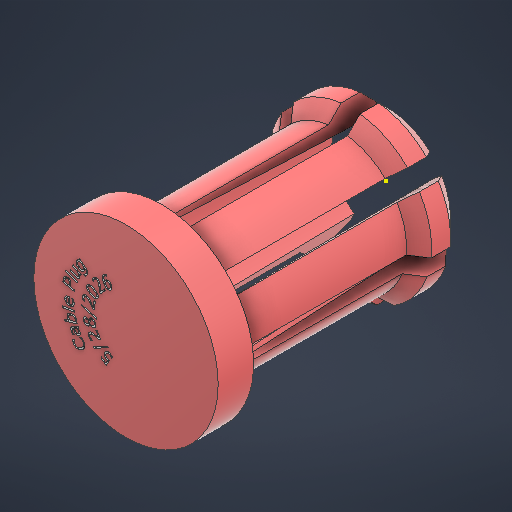
# Autodesk Inventor part: WirePlugs
Saved by Autodesk Inventor 2026.2 (Build 302298000, 298)
## iProperties
Created: 2026-05-27
Part Number: WirePlugs
Material: Generic
Document SubType Name: Modeling
Designer: mayhe
Density: 1 g/cm^3
Appearance: Default
Author: mayhe
Autodesk Inventor part; units mm, degrees
ref_plane "YZ Plane" through (0, 0, 0) normal (1, 0, 0) x (0, 1, 0)
ref_plane "XZ Plane" through (0, 0, 0) normal (0, 1, 0) x (-1, 0, 0)
ref_plane "XY Plane" through (0, 0, 0) normal (0, 0, 1) x (1, 0, 0)
sketch "Sketch1" plane through (0, 0, 0) normal (0, 0, 1) x (1, 0, 0)
  circle A0 centre (0, 0) radius 19.5
  dimension "d0" = 39
  constraints: 1 centre point, 1 coincident
  measures "d0" diameter of A0
extrude "Body" add sketch "Sketch1" along normal mid plane 55
sketch "Sketch2" plane through (0, 0, -27.5) normal (0, 0, -1) x (-1, 0, 0)
  point P0 (0, 0)
sketch "Sketch3" plane through (0, 0, 0) normal (1, 0, 0) x (0, 1, 0)
  line L0 (19.5, 20) -> (14.5, 20)
  line L1 (14.5, 20) -> (14.5, -20)
  line L2 (14.5, -20) -> (17.15, -20)
  line L3 (17.15, -20) -> (17.15, -27.5)
  line L4 (-19.5, -27.5) -> (19.5, -27.5) projected
  line L5 (19.5, 20) -> (19.5, -27.5)
  line L6 (17.15, -27.5) -> (19.5, -27.5)
  line L7 (0, -38.5) -> (0, 38.5) projected
  line L8 (19.5, 27.5) -> (-19.5, 27.5) projected
  point P0 (0, 0)
  dimension "d4" = 5
  dimension "d5" = 40
  dimension "d6" = 2.65
  dimension "d27" = 7.5
  constraints: 12 end point, 3 perpendicular, 1 collinear, 1 horizontal, 1 point on line
  measures "d4" distance of L0.start L0.end
  measures "d5" distance of L0.end L1.end
  measures "d6" distance of L1.end L2.end
  measures "d27" distance from line of L8 L0.start
revolve "Revolution1" cut sketch "Sketch3" angle 360 about axis through (0, 0, -10) along (0, 0, 1)
chamfer "Chamfer1" distance 3.5 angle 45 1 edges at (0, -17.15, -27.5)
chamfer "Chamfer2" distance 2.65 angle 45 1 edges at (0, -14.5, -20)
sketch "Sketch4" plane through (0, 0, -27.5) normal (0, 0, -1) x (-1, 0, 0)
  circle A0 centre (0, 0) radius 11.5
  dimension "d14" = 23
  constraints: 1 centre point, 1 coincident
  measures "d14" diameter of A0
extrude "Extrusion2" cut sketch "Sketch4" against normal up to surface (47.5 mm away) draft 2.5
sketch "Sketch5" plane through (0, 0, -27.5) normal (0, 0, -1) x (-1, 0, 0)
  line L0 (-2, 18.114) -> (2, 18.114)
  line L1 (2, 18.114) -> (2, 9.186)
  line L2 (2, 9.186) -> (-2, 9.186)
  line L3 (-2, 9.186) -> (-2, 18.114)
  circle A0 centre (0, 0) radius 13.65 projected
  line L4 (-2, 18.114) -> (2, 9.186) construction
  line L5 (2, 18.114) -> (-2, 9.186) construction
  line L6 (-15.4091, 9.7302) -> (-12.9151, 12.8576)
  line L7 (-12.9151, 12.8576) -> (-8.4289, 4.1637) construction
  line L8 (-12.9151, 12.8576) -> (-5.9349, 7.291)
  line L9 (-15.4091, 9.7302) -> (-5.9349, 7.291) construction
  line L10 (-8.4289, 4.1637) -> (-15.4091, 9.7302)
  line L11 (-5.9349, 7.291) -> (-8.4289, 4.1637)
  line L12 (-17.2148, -5.9806) -> (-18.1049, -2.0809)
  line L13 (-18.1049, -2.0809) -> (-8.5106, -3.9939) construction
  line L14 (-18.1049, -2.0809) -> (-9.4007, -0.0942)
  line L15 (-17.2148, -5.9806) -> (-9.4007, -0.0942) construction
  line L16 (-8.5106, -3.9939) -> (-17.2148, -5.9806)
  line L17 (-9.4007, -0.0942) -> (-8.5106, -3.9939)
  line L18 (-6.0574, -17.1879) -> (-9.6613, -15.4524)
  line L19 (-9.6613, -15.4524) -> (-2.1837, -9.144) construction
  line L20 (-9.6613, -15.4524) -> (-5.7876, -7.4085)
  line L21 (-6.0574, -17.1879) -> (-5.7876, -7.4085) construction
  line L22 (-2.1837, -9.144) -> (-6.0574, -17.1879)
  line L23 (-5.7876, -7.4085) -> (-2.1837, -9.144)
  line L24 (9.6613, -15.4524) -> (6.0574, -17.1879)
  line L25 (6.0574, -17.1879) -> (5.7876, -7.4085) construction
  line L26 (6.0574, -17.1879) -> (2.1837, -9.144)
  line L27 (9.6613, -15.4524) -> (2.1837, -9.144) construction
  line L28 (5.7876, -7.4085) -> (9.6613, -15.4524)
  line L29 (2.1837, -9.144) -> (5.7876, -7.4085)
  line L30 (18.1049, -2.0809) -> (17.2148, -5.9806)
  line L31 (17.2148, -5.9806) -> (9.4007, -0.0942) construction
  line L32 (17.2148, -5.9806) -> (8.5106, -3.9939)
  line L33 (18.1049, -2.0809) -> (8.5106, -3.9939) construction
  line L34 (9.4007, -0.0942) -> (18.1049, -2.0809)
  line L35 (8.5106, -3.9939) -> (9.4007, -0.0942)
  line L36 (12.9151, 12.8576) -> (15.4091, 9.7302)
  line L37 (15.4091, 9.7302) -> (5.9349, 7.291) construction
  line L38 (15.4091, 9.7302) -> (8.4289, 4.1637)
  line L39 (12.9151, 12.8576) -> (8.4289, 4.1637) construction
  line L40 (5.9349, 7.291) -> (12.9151, 12.8576)
  line L41 (8.4289, 4.1637) -> (5.9349, 7.291)
  point P0 (0, 13.65)
  point P1 (-10.672, 8.5106)
  point P2 (-13.3078, -3.0374)
  point P3 (-5.9225, -12.2982)
  point P4 (5.9225, -12.2982)
  point P5 (13.3078, -3.0374)
  point P6 (10.672, 8.5106)
  dimension "d17" = 4
  dimension "d20" = 360
  constraints: 84 end point, 2 midpoint, 2 parallel, 1 horizontal, 1 perpendicular, 1 vertical alignment, 79 other
  measures "d17" distance of L1.end L2.end
extrude "Extrusion3" cut sketch "Sketch5" against normal up to surface (47.5 mm away) contours L0 L1 A0 L3 | A0 L1 L2 L3 | L8 L11 L10 A0 | A0 L10 L6 L8 | L40 L36 L38 A0 | A0 L38 L41 L40 | L14 L17 L16 A0 | A0 L16 L12 L14 | L34 L30 L32 A0 | A0 L32 L35 L34 | L20 L23 L22 A0 | A0 L22 L18 L20 | L28 L24 L26 A0 | A0 L26 L29 L28
chamfer "Chamfer3" distance 1 angle 45 14 edges at (-2, 13.8936, 20) (2, 13.8936, 20) (9.6155, 10.2262, 20) (12.1094, 7.0988, 20) (13.9903, -1.1418, 20) (13.1002, -5.0415, 20) (7.8301, -11.6499, 20) (4.2263, -13.3854, 20) (-4.2263, -13.3854, 20) (-7.8301, -11.6499, 20) (-13.1002, -5.0415, 20) (-13.9903, -1.1418, 20) (-12.1094, 7.0988, 20) (-9.6155, 10.2262, 20)
sketch "Sketch6" plane through (0, 0, 27.5) normal (0, 0, 1) x (1, 0, 0)
  circle A0 centre (0, 0) radius 11
  spline S0 degree 2 poles (-8.9107, -6.3753) (-8.7634, -6.5735) (-8.6478, -7.0083) (-8.6908, -7.23) knots 0 0 0 1 2 2 2
  spline S1 degree 2 poles (-8.6908, -7.23) (-8.732, -7.4505) (-9.029, -7.8791) (-9.2866, -8.0707) knots 0 0 0 1 2 2 2
  spline S2 degree 2 poles (-9.2866, -8.0707) (-9.5427, -8.261) (-10.0196, -8.413) (-10.2521, -8.3935) knots 0 0 0 1 2 2 2
  spline S3 degree 2 poles (-10.2521, -8.3935) (-10.4801, -8.3732) (-10.8719, -8.1464) (-11.0254, -7.94) knots 0 0 0 1 2 2 2
  spline S4 degree 2 poles (-11.0254, -7.94) (-11.1016, -7.8375) (-11.2057, -7.6354) (-11.2391, -7.5422) knots 0 0 0 1 2 2 2
  spline S5 degree 2 poles (-11.2391, -7.5422) (-11.2667, -7.4602) (-11.3075, -7.2776) (-11.3216, -7.1829) knots 0 0 0 1 2 2 2
  line L0 (-11.3216, -7.1829) -> (-10.9945, -6.9397)
  line L1 (-10.9945, -6.9397) -> (-10.9785, -6.9612)
  spline S6 degree 2 poles (-10.9785, -6.9612) (-10.9846, -7.0221) (-10.9935, -7.2032) (-10.978, -7.3173) knots 0 0 0 1 2 2 2
  spline S7 degree 2 poles (-10.978, -7.3173) (-10.9632, -7.4269) (-10.8814, -7.6507) (-10.7929, -7.7697) knots 0 0 0 1 2 2 2
  spline S8 degree 2 poles (-10.7929, -7.7697) (-10.6959, -7.9002) (-10.4154, -8.0532) (-10.2479, -8.0646) knots 0 0 0 1 2 2 2
  spline S9 degree 2 poles (-10.2479, -8.0646) (-10.0799, -8.0731) (-9.6932, -7.9344) (-9.4967, -7.7882) knots 0 0 0 1 2 2 2
  spline S10 degree 2 poles (-9.4967, -7.7882) (-9.2869, -7.6322) (-9.0595, -7.3067) (-9.0206, -7.1418) knots 0 0 0 1 2 2 2
  spline S11 degree 2 poles (-9.0206, -7.1418) (-8.9837, -6.981) (-9.052, -6.6753) (-9.1478, -6.5464) knots 0 0 0 1 2 2 2
  spline S12 degree 2 poles (-9.1478, -6.5464) (-9.235, -6.4291) (-9.4414, -6.2723) (-9.542, -6.2266) knots 0 0 0 1 2 2 2
  spline S13 degree 2 poles (-9.542, -6.2266) (-9.6403, -6.1842) (-9.8117, -6.1398) (-9.8665, -6.1318) knots 0 0 0 1 2 2 2
  line L2 (-9.8665, -6.1318) -> (-9.8812, -6.1119)
  line L3 (-9.8812, -6.1119) -> (-9.5574, -5.8712)
  spline S14 degree 2 poles (-9.5574, -5.8712) (-9.4757, -5.9156) (-9.3295, -5.9915) (-9.2404, -6.0561) knots 0 0 0 1 2 2 2
  spline S15 degree 2 poles (-9.2404, -6.0561) (-9.1444, -6.1232) (-9.0016, -6.2531) (-8.9107, -6.3753) knots 0 0 0 1 2 2 2
  spline S16 degree 2 poles (-10.1998, -4.646) (-10.1566, -4.6682) (-10.0058, -4.7404) (-9.9507, -4.782) knots 0 0 0 1 2 2 2
  spline S17 degree 2 poles (-9.9507, -4.782) (-9.8726, -4.8374) (-9.7596, -4.9583) (-9.6955, -5.0873) knots 0 0 0 1 2 2 2
  spline S18 degree 2 poles (-9.6955, -5.0873) (-9.6433, -5.1924) (-9.6283, -5.4216) (-9.6644, -5.5292) knots 0 0 0 1 2 2 2
  spline S19 degree 2 poles (-9.6644, -5.5292) (-9.7006, -5.6322) (-9.8658, -5.8178) (-9.9801, -5.8745) knots 0 0 0 1 2 2 2
  spline S20 degree 2 poles (-9.9801, -5.8745) (-10.1571, -5.9625) (-10.482, -5.9377) (-10.6345, -5.8112) knots 0 0 0 1 2 2 2
  spline S21 degree 2 poles (-10.6345, -5.8112) (-10.7723, -5.7004) (-11.0162, -5.3343) (-11.1417, -5.114) knots 0 0 0 1 2 2 2
  line L4 (-11.1417, -5.114) -> (-11.197, -5.1415)
  spline S22 degree 2 poles (-11.197, -5.1415) (-11.2966, -5.191) (-11.3899, -5.3132) (-11.3974, -5.3859) knots 0 0 0 1 2 2 2
  spline S23 degree 2 poles (-11.3974, -5.3859) (-11.405, -5.4586) (-11.3483, -5.6281) (-11.3062, -5.7129) knots 0 0 0 1 2 2 2
  spline S24 degree 2 poles (-11.3062, -5.7129) (-11.2567, -5.8124) (-11.064, -6.0522) (-10.94, -6.1584) knots 0 0 0 1 2 2 2
  line L5 (-10.94, -6.1584) -> (-10.9318, -6.175)
  line L6 (-10.9318, -6.175) -> (-11.2249, -6.3206)
  spline S25 degree 2 poles (-11.2249, -6.3206) (-11.2864, -6.2523) (-11.4891, -5.983) (-11.5615, -5.8374) knots 0 0 0 1 2 2 2
  spline S26 degree 2 poles (-11.5615, -5.8374) (-11.6494, -5.6605) (-11.7141, -5.3915) (-11.6898, -5.2599) knots 0 0 0 1 2 2 2
  spline S27 degree 2 poles (-11.6898, -5.2599) (-11.6665, -5.1311) (-11.4892, -4.9281) (-11.3289, -4.8484) knots 0 0 0 1 2 2 2
  line L7 (-11.3289, -4.8484) -> (-10.162, -4.2687)
  line L8 (-10.162, -4.2687) -> (-10.0191, -4.5563)
  line L9 (-10.0191, -4.5563) -> (-10.1998, -4.646)
  line L10 (-10.4394, -4.7651) -> (-10.9132, -5.0005)
  spline S28 degree 2 poles (-10.9132, -5.0005) (-10.8527, -5.0991) (-10.6665, -5.3951) (-10.5885, -5.4781) knots 0 0 0 1 2 2 2
  spline S29 degree 2 poles (-10.5885, -5.4781) (-10.4967, -5.575) (-10.2769, -5.652) (-10.1479, -5.5878) knots 0 0 0 1 2 2 2
  spline S30 degree 2 poles (-10.1479, -5.5878) (-10.0004, -5.5146) (-9.9335, -5.2745) (-10.0123, -5.116) knots 0 0 0 1 2 2 2
  spline S31 degree 2 poles (-10.0123, -5.116) (-10.0791, -4.9814) (-10.3052, -4.8179) (-10.4394, -4.7651) knots 0 0 0 1 2 2 2
  spline S32 degree 2 poles (-11.7296, -2.6033) (-11.2819, -2.4695) (-10.606, -2.7401) (-10.5081, -3.0675) knots 0 0 0 1 2 2 2
  spline S33 degree 2 poles (-10.5081, -3.0675) (-10.4639, -3.2154) (-10.4738, -3.4482) (-10.5063, -3.5697) knots 0 0 0 1 2 2 2
  line L11 (-10.5063, -3.5697) -> (-10.4156, -3.564)
  line L12 (-10.4156, -3.564) -> (-10.3295, -3.852)
  line L13 (-10.3295, -3.852) -> (-12.8716, -4.6117)
  line L14 (-12.8716, -4.6117) -> (-12.9636, -4.3041)
  line L15 (-12.9636, -4.3041) -> (-12.0564, -4.0329)
  spline S34 degree 2 poles (-12.0564, -4.0329) (-12.1957, -3.9478) (-12.4145, -3.7189) (-12.4658, -3.5473) knots 0 0 0 1 2 2 2
  spline S35 degree 2 poles (-12.4658, -3.5473) (-12.5583, -3.2377) (-12.1694, -2.7348) (-11.7296, -2.6033) knots 0 0 0 1 2 2 2
  spline S36 degree 2 poles (-11.611, -2.9138) (-11.9384, -3.0116) (-12.2181, -3.3122) (-12.1521, -3.5331) knots 0 0 0 1 2 2 2
  spline S37 degree 2 poles (-12.1521, -3.5331) (-12.115, -3.6573) (-11.92, -3.8783) (-11.798, -3.9557) knots 0 0 0 1 2 2 2
  line L16 (-11.798, -3.9557) -> (-10.7508, -3.6427)
  spline S38 degree 2 poles (-10.7508, -3.6427) (-10.7284, -3.5093) (-10.7347, -3.3157) (-10.7665, -3.2092) knots 0 0 0 1 2 2 2
  spline S39 degree 2 poles (-10.7665, -3.2092) (-10.8367, -2.9745) (-11.2501, -2.8059) (-11.611, -2.9138) knots 0 0 0 1 2 2 2
  line L17 (-10.8743, -1.6658) -> (-10.8211, -1.9824)
  line L18 (-10.8211, -1.9824) -> (-13.4376, -2.4224)
  line L19 (-13.4376, -2.4224) -> (-13.4908, -2.1057)
  line L20 (-13.4908, -2.1057) -> (-10.8743, -1.6658)
  spline S40 degree 2 poles (-10.9513, -0.3734) (-10.9299, -0.8299) (-11.4183, -1.3556) (-11.8912, -1.3778) knots 0 0 0 1 2 2 2
  spline S41 degree 2 poles (-11.8912, -1.3778) (-12.3558, -1.3997) (-12.9298, -0.9383) (-12.9482, -0.5456) knots 0 0 0 1 2 2 2
  spline S42 degree 2 poles (-12.9482, -0.5456) (-12.9565, -0.3687) (-12.8666, -0.0905) (-12.7623, 0.0154) knots 0 0 0 1 2 2 2
  spline S43 degree 2 poles (-12.7623, 0.0154) (-12.6582, 0.1233) (-12.3487, 0.2471) (-12.1205, 0.2578) knots 0 0 0 1 2 2 2
  line L21 (-12.1205, 0.2578) -> (-11.9457, 0.266)
  line L22 (-11.9457, 0.266) -> (-11.8838, -1.0519)
  spline S44 degree 2 poles (-11.8838, -1.0519) (-11.5528, -1.0364) (-11.2168, -0.6868) (-11.2308, -0.3907) knots 0 0 0 1 2 2 2
  spline S45 degree 2 poles (-11.2308, -0.3907) (-11.2357, -0.2858) (-11.2925, -0.0845) (-11.3334, -0.004) knots 0 0 0 1 2 2 2
  spline S46 degree 2 poles (-11.3334, -0.004) (-11.3786, 0.0804) (-11.4562, 0.1963) (-11.4909, 0.2338) knots 0 0 0 1 2 2 2
  line L23 (-11.4909, 0.2338) -> (-11.4918, 0.2523)
  line L24 (-11.4918, 0.2523) -> (-11.1422, 0.2688)
  spline S47 degree 2 poles (-11.1422, 0.2688) (-11.117, 0.2143) (-11.0433, 0.0488) (-11.0217, -0.0161) knots 0 0 0 1 2 2 2
  spline S48 degree 2 poles (-11.0217, -0.0161) (-10.9906, -0.1074) (-10.9567, -0.2583) (-10.9513, -0.3734) knots 0 0 0 1 2 2 2
  spline S49 degree 2 poles (-12.1757, -0.058) (-12.3051, -0.0682) (-12.4917, -0.1305) (-12.553, -0.1849) knots 0 0 0 1 2 2 2
  spline S50 degree 2 poles (-12.553, -0.1849) (-12.6224, -0.2438) (-12.6902, -0.4222) (-12.6842, -0.5517) knots 0 0 0 1 2 2 2
  spline S51 degree 2 poles (-12.6842, -0.5517) (-12.6782, -0.6792) (-12.5937, -0.8545) (-12.5162, -0.925) knots 0 0 0 1 2 2 2
  spline S52 degree 2 poles (-12.5162, -0.925) (-12.4367, -0.9934) (-12.2503, -1.0588) (-12.1285, -1.0634) knots 0 0 0 1 2 2 2
  line L25 (-12.1285, -1.0634) -> (-12.1757, -0.058)
  spline S53 degree 2 poles (-12.2596, 3.7005) (-12.099, 3.6641) (-11.8359, 3.4841) (-11.7587, 3.359) knots 0 0 0 1 2 2 2
  spline S54 degree 2 poles (-11.7587, 3.359) (-11.6614, 3.2019) (-11.6096, 2.825) (-11.6696, 2.56) knots 0 0 0 1 2 2 2
  line L26 (-11.6696, 2.56) -> (-11.7328, 2.281)
  line L27 (-11.7328, 2.281) -> (-10.8094, 2.0717)
  line L28 (-10.8094, 2.0717) -> (-10.884, 1.7425)
  line L29 (-10.884, 1.7425) -> (-13.3612, 2.3039)
  line L30 (-13.3612, 2.3039) -> (-13.2202, 2.9262)
  spline S55 degree 2 poles (-13.2202, 2.9262) (-13.1702, 3.147) (-13.0278, 3.4398) (-12.9187, 3.5396) knots 0 0 0 1 2 2 2
  spline S56 degree 2 poles (-12.9187, 3.5396) (-12.7929, 3.6567) (-12.4664, 3.7473) (-12.2596, 3.7005) knots 0 0 0 1 2 2 2
  spline S57 degree 2 poles (-12.3274, 3.3549) (-12.4558, 3.384) (-12.6646, 3.3385) (-12.7453, 3.2618) knots 0 0 0 1 2 2 2
  spline S58 degree 2 poles (-12.7453, 3.2618) (-12.8152, 3.1953) (-12.9047, 2.9961) (-12.9397, 2.8415) knots 0 0 0 1 2 2 2
  line L31 (-12.9397, 2.8415) -> (-13.0016, 2.5685)
  line L32 (-13.0016, 2.5685) -> (-12.0139, 2.3447)
  line L33 (-12.0139, 2.3447) -> (-11.9629, 2.5695)
  spline S59 degree 2 poles (-11.9629, 2.5695) (-11.9175, 2.7703) (-11.9257, 3.0317) (-11.9919, 3.1311) knots 0 0 0 1 2 2 2
  spline S60 degree 2 poles (-11.9919, 3.1311) (-12.0493, 3.2223) (-12.2089, 3.3281) (-12.3274, 3.3549) knots 0 0 0 1 2 2 2
  line L34 (-10.2918, 3.8865) -> (-10.4008, 3.5845)
  line L35 (-10.4008, 3.5845) -> (-12.8964, 4.4855)
  line L36 (-12.8964, 4.4855) -> (-12.7873, 4.7875)
  line L37 (-12.7873, 4.7875) -> (-10.2918, 3.8865)
  line L38 (-9.4657, 5.6523) -> (-9.6115, 5.3662)
  line L39 (-9.6115, 5.3662) -> (-9.7986, 5.4615)
  spline S61 degree 2 poles (-9.7986, 5.4615) (-9.7503, 5.2706) (-9.7515, 4.9732) (-9.8263, 4.8265) knots 0 0 0 1 2 2 2
  spline S62 degree 2 poles (-9.8263, 4.8265) (-9.8823, 4.7165) (-10.0556, 4.5576) (-10.1709, 4.5262) knots 0 0 0 1 2 2 2
  spline S63 degree 2 poles (-10.1709, 4.5262) (-10.2872, 4.493) (-10.5685, 4.5347) (-10.741, 4.6225) knots 0 0 0 1 2 2 2
  line L40 (-10.741, 4.6225) -> (-11.8433, 5.1839)
  line L41 (-11.8433, 5.1839) -> (-11.6976, 5.47)
  line L42 (-11.6976, 5.47) -> (-10.7291, 4.9768)
  spline S64 degree 2 poles (-10.7291, 4.9768) (-10.5934, 4.9077) (-10.4052, 4.8372) (-10.3214, 4.8385) knots 0 0 0 1 2 2 2
  spline S65 degree 2 poles (-10.3214, 4.8385) (-10.2377, 4.8397) (-10.1164, 4.9281) (-10.0594, 5.04) knots 0 0 0 1 2 2 2
  spline S66 degree 2 poles (-10.0594, 5.04) (-10.0062, 5.1445) (-10.0049, 5.4418) (-10.0407, 5.5848) knots 0 0 0 1 2 2 2
  line L43 (-10.0407, 5.5848) -> (-11.3099, 6.2312)
  line L44 (-11.3099, 6.2312) -> (-11.1642, 6.5173)
  line L45 (-11.1642, 6.5173) -> (-9.4657, 5.6523)
  spline S67 degree 2 poles (-8.9354, 5.9154) (-8.904, 5.933) (-8.7922, 6.0059) (-8.729, 6.0588) knots 0 0 0 1 2 2 2
  spline S68 degree 2 poles (-8.729, 6.0588) (-8.6576, 6.1158) (-8.5457, 6.2196) (-8.4924, 6.2902) knots 0 0 0 1 2 2 2
  spline S69 degree 2 poles (-8.4924, 6.2902) (-8.4031, 6.4085) (-8.3414, 6.6198) (-8.3625, 6.708) knots 0 0 0 1 2 2 2
  spline S70 degree 2 poles (-8.3625, 6.708) (-8.3849, 6.7945) (-8.505, 6.9394) (-8.5986, 7.0102) knots 0 0 0 1 2 2 2
  line L46 (-8.5986, 7.0102) -> (-8.7317, 7.1106)
  spline S71 degree 2 poles (-8.7317, 7.1106) (-8.7195, 6.9389) (-8.7842, 6.6757) (-8.8971, 6.5262) knots 0 0 0 1 2 2 2
  spline S72 degree 2 poles (-8.8971, 6.5262) (-9.0931, 6.2667) (-9.7111, 6.2511) (-10.0741, 6.5252) knots 0 0 0 1 2 2 2
  spline S73 degree 2 poles (-10.0741, 6.5252) (-10.2629, 6.6679) (-10.4747, 6.9955) (-10.5112, 7.1623) knots 0 0 0 1 2 2 2
  spline S74 degree 2 poles (-10.5112, 7.1623) (-10.5436, 7.3209) (-10.4729, 7.6364) (-10.3787, 7.7613) knots 0 0 0 1 2 2 2
  spline S75 degree 2 poles (-10.3787, 7.7613) (-10.2893, 7.8795) (-10.1032, 8.0098) (-9.9866, 8.0584) knots 0 0 0 1 2 2 2
  line L47 (-9.9866, 8.0584) -> (-10.0395, 8.1216)
  line L48 (-10.0395, 8.1216) -> (-9.8571, 8.363)
  line L49 (-9.8571, 8.363) -> (-8.5102, 7.3458)
  spline S76 degree 2 poles (-8.5102, 7.3458) (-8.1226, 7.053) (-8.0156, 6.4434) (-8.2773, 6.0968) knots 0 0 0 1 2 2 2
  spline S77 degree 2 poles (-8.2773, 6.0968) (-8.3617, 5.9851) (-8.574, 5.7792) (-8.6792, 5.7013) knots 0 0 0 1 2 2 2
  line L50 (-8.6792, 5.7013) -> (-8.9453, 5.9023)
  line L51 (-8.9453, 5.9023) -> (-8.9354, 5.9154)
  line L52 (-8.9419, 7.2694) -> (-9.778, 7.9009)
  spline S78 degree 2 poles (-9.778, 7.9009) (-9.8959, 7.8403) (-10.0569, 7.7091) (-10.1177, 7.6286) knots 0 0 0 1 2 2 2
  spline S79 degree 2 poles (-10.1177, 7.6286) (-10.2641, 7.4348) (-10.147, 6.9956) (-9.8793, 6.7934) knots 0 0 0 1 2 2 2
  spline S80 degree 2 poles (-9.8793, 6.7934) (-9.6263, 6.6023) (-9.2341, 6.5718) (-9.0902, 6.7623) knots 0 0 0 1 2 2 2
  spline S81 degree 2 poles (-9.0902, 6.7623) (-9.0145, 6.8625) (-8.9346, 7.1323) (-8.9419, 7.2694) knots 0 0 0 1 2 2 2
  spline S82 degree 2 poles (-4.4923, -6.1203) (-4.3995, -5.9624) (-4.1398, -5.7521) (-3.9892, -5.707) knots 0 0 0 1 2 2 2
  spline S83 degree 2 poles (-3.9892, -5.707) (-3.8385, -5.6618) (-3.4956, -5.7081) (-3.3253, -5.8082) knots 0 0 0 1 2 2 2
  spline S84 degree 2 poles (-3.3253, -5.8082) (-3.1691, -5.9) (-2.9046, -6.1486) (-2.8251, -6.2693) knots 0 0 0 1 2 2 2
  line L53 (-2.8251, -6.2693) -> (-3.0076, -6.5799)
  line L54 (-3.0076, -6.5799) -> (-3.0289, -6.5674)
  spline S85 degree 2 poles (-3.0289, -6.5674) (-3.048, -6.5227) (-3.1365, -6.3848) (-3.1961, -6.3115) knots 0 0 0 1 2 2 2
  spline S86 degree 2 poles (-3.1961, -6.3115) (-3.2653, -6.2303) (-3.3892, -6.1121) (-3.4797, -6.0589) knots 0 0 0 1 2 2 2
  spline S87 degree 2 poles (-3.4797, -6.0589) (-3.5685, -6.0067) (-3.7728, -5.9726) (-3.8738, -6.0063) knots 0 0 0 1 2 2 2
  spline S88 degree 2 poles (-3.8738, -6.0063) (-3.9674, -6.0397) (-4.1264, -6.1802) (-4.1953, -6.2973) knots 0 0 0 1 2 2 2
  spline S89 degree 2 poles (-4.1953, -6.2973) (-4.2641, -6.4144) (-4.2878, -6.601) (-4.2567, -6.6862) knots 0 0 0 1 2 2 2
  spline S90 degree 2 poles (-4.2567, -6.6862) (-4.2269, -6.7777) (-4.0695, -6.9323) (-3.9577, -6.998) knots 0 0 0 1 2 2 2
  spline S91 degree 2 poles (-3.9577, -6.998) (-3.837, -7.0689) (-3.5755, -7.1725) (-3.4934, -7.1993) knots 0 0 0 1 2 2 2
  line L55 (-3.4934, -7.1993) -> (-4.1567, -8.3279)
  line L56 (-4.1567, -8.3279) -> (-5.3581, -7.6218)
  line L57 (-5.3581, -7.6218) -> (-5.2069, -7.3645)
  line L58 (-5.2069, -7.3645) -> (-4.2876, -7.9047)
  line L59 (-4.2876, -7.9047) -> (-3.9445, -7.3209)
  spline S92 degree 2 poles (-3.9445, -7.3209) (-4.0019, -7.2967) (-4.108, -7.2415) (-4.1506, -7.2165) knots 0 0 0 1 2 2 2
  spline S93 degree 2 poles (-4.1506, -7.2165) (-4.3191, -7.1174) (-4.5193, -6.9258) (-4.5778, -6.7816) knots 0 0 0 1 2 2 2
  spline S94 degree 2 poles (-4.5778, -6.7816) (-4.638, -6.6363) (-4.6092, -6.3191) (-4.4923, -6.1203) knots 0 0 0 1 2 2 2
  line L60 (-6.957, -6.346) -> (-4.0116, -4.7384)
  line L61 (-4.0116, -4.7384) -> (-3.8048, -4.9391)
  line L62 (-3.8048, -4.9391) -> (-6.7472, -6.5496)
  line L63 (-6.7472, -6.5496) -> (-6.957, -6.346)
  line L64 (-6.1357, -2.9151) -> (-5.3018, -4.2411)
  line L65 (-5.3018, -4.2411) -> (-5.6067, -4.4329)
  spline S95 degree 2 poles (-5.6067, -4.4329) (-5.8307, -4.3744) (-6.2399, -4.2767) (-6.4508, -4.2391) knots 0 0 0 1 2 2 2
  spline S96 degree 2 poles (-6.4508, -4.2391) (-6.8753, -4.1632) (-7.3123, -4.1876) (-7.4848, -4.2961) knots 0 0 0 1 2 2 2
  spline S97 degree 2 poles (-7.4848, -4.2961) (-7.5754, -4.3531) (-7.6762, -4.4943) (-7.688, -4.5722) knots 0 0 0 1 2 2 2
  spline S98 degree 2 poles (-7.688, -4.5722) (-7.6998, -4.6501) (-7.6601, -4.8099) (-7.6097, -4.8901) knots 0 0 0 1 2 2 2
  spline S99 degree 2 poles (-7.6097, -4.8901) (-7.5615, -4.9668) (-7.4245, -5.0995) (-7.35, -5.1523) knots 0 0 0 1 2 2 2
  spline S100 degree 2 poles (-7.35, -5.1523) (-7.2872, -5.1979) (-7.1463, -5.2674) (-7.1, -5.2869) knots 0 0 0 1 2 2 2
  line L66 (-7.1, -5.2869) -> (-7.0901, -5.3026)
  line L67 (-7.0901, -5.3026) -> (-7.3968, -5.4954)
  spline S101 degree 2 poles (-7.3968, -5.4954) (-7.4962, -5.4339) (-7.7821, -5.1688) (-7.872, -5.0259) knots 0 0 0 1 2 2 2
  spline S102 degree 2 poles (-7.872, -5.0259) (-8.0616, -4.7244) (-7.9564, -4.1841) (-7.6846, -4.0132) knots 0 0 0 1 2 2 2
  spline S103 degree 2 poles (-7.6846, -4.0132) (-7.5574, -3.9332) (-7.3075, -3.8588) (-7.1841, -3.8541) knots 0 0 0 1 2 2 2
  spline S104 degree 2 poles (-7.1841, -3.8541) (-7.0571, -3.8472) (-6.7771, -3.8826) (-6.6356, -3.9104) knots 0 0 0 1 2 2 2
  spline S105 degree 2 poles (-6.6356, -3.9104) (-6.402, -3.9531) (-5.8756, -4.0865) (-5.7208, -4.1277) knots 0 0 0 1 2 2 2
  line L68 (-5.7208, -4.1277) -> (-6.3848, -3.0718)
  line L69 (-6.3848, -3.0718) -> (-6.1357, -2.9151)
  spline S106 degree 2 poles (-6.4265, -1.8528) (-6.374, -2.0347) (-6.3967, -2.3647) (-6.4673, -2.4986) knots 0 0 0 1 2 2 2
  spline S107 degree 2 poles (-6.4673, -2.4986) (-6.5366, -2.63) (-6.7748, -2.8143) (-6.9271, -2.8582) knots 0 0 0 1 2 2 2
  spline S108 degree 2 poles (-6.9271, -2.8582) (-7.1248, -2.9153) (-7.5181, -2.7994) (-7.6752, -2.6262) knots 0 0 0 1 2 2 2
  line L70 (-7.6752, -2.6262) -> (-7.6851, -2.6291)
  spline S109 degree 2 poles (-7.6851, -2.6291) (-7.738, -2.8393) (-7.937, -3.0852) (-8.1229, -3.1388) knots 0 0 0 1 2 2 2
  spline S110 degree 2 poles (-8.1229, -3.1388) (-8.3978, -3.218) (-8.8855, -2.9087) (-8.9778, -2.5883) knots 0 0 0 1 2 2 2
  spline S111 degree 2 poles (-8.9778, -2.5883) (-9.0736, -2.2561) (-8.8413, -1.7542) (-8.5683, -1.6755) knots 0 0 0 1 2 2 2
  spline S112 degree 2 poles (-8.5683, -1.6755) (-8.4042, -1.6282) (-8.0285, -1.7277) (-7.8856, -1.8814) knots 0 0 0 1 2 2 2
  line L71 (-7.8856, -1.8814) -> (-7.8757, -1.8786)
  spline S113 degree 2 poles (-7.8757, -1.8786) (-7.8384, -1.6365) (-7.6169, -1.3348) (-7.3914, -1.2698) knots 0 0 0 1 2 2 2
  spline S114 degree 2 poles (-7.3914, -1.2698) (-7.0789, -1.1797) (-6.5245, -1.5126) (-6.4265, -1.8528) knots 0 0 0 1 2 2 2
  spline S115 degree 2 poles (-7.2629, -1.5969) (-7.4132, -1.6402) (-7.557, -1.8102) (-7.5995, -2.0046) knots 0 0 0 1 2 2 2
  spline S116 degree 2 poles (-7.5995, -2.0046) (-7.6151, -2.0691) (-7.6347, -2.2761) (-7.6486, -2.4065) knots 0 0 0 1 2 2 2
  spline S117 degree 2 poles (-7.6486, -2.4065) (-7.5208, -2.5153) (-7.2141, -2.5833) (-7.046, -2.5348) knots 0 0 0 1 2 2 2
  spline S118 degree 2 poles (-7.046, -2.5348) (-6.8245, -2.4709) (-6.6127, -2.1207) (-6.6709, -1.9189) knots 0 0 0 1 2 2 2
  spline S119 degree 2 poles (-6.6709, -1.9189) (-6.7302, -1.7133) (-7.0493, -1.5353) (-7.2629, -1.5969) knots 0 0 0 1 2 2 2
  spline S120 degree 2 poles (-8.472, -1.9948) (-8.6362, -2.0421) (-8.7924, -2.3249) (-8.736, -2.5207) knots 0 0 0 1 2 2 2
  spline S121 degree 2 poles (-8.736, -2.5207) (-8.6846, -2.6987) (-8.4233, -2.8697) (-8.2552, -2.8213) knots 0 0 0 1 2 2 2
  spline S122 degree 2 poles (-8.2552, -2.8213) (-8.1345, -2.7865) (-8, -2.6213) (-7.9664, -2.4853) knots 0 0 0 1 2 2 2
  spline S123 degree 2 poles (-7.9664, -2.4853) (-7.953, -2.4278) (-7.9165, -2.1902) (-7.9134, -2.0972) knots 0 0 0 1 2 2 2
  spline S124 degree 2 poles (-7.9134, -2.0972) (-8.0632, -1.9862) (-8.3237, -1.952) (-8.472, -1.9948) knots 0 0 0 1 2 2 2
  line L72 (-9.4148, 0.1814) -> (-6.1713, -0.6785)
  line L73 (-6.1713, -0.6785) -> (-6.1593, -0.9664)
  line L74 (-6.1593, -0.9664) -> (-9.4026, -0.1107)
  line L75 (-9.4026, -0.1107) -> (-9.4148, 0.1814)
  line L76 (-6.4583, 2.106) -> (-6.7654, 0.57)
  line L77 (-6.7654, 0.57) -> (-7.1186, 0.6407)
  spline S125 degree 2 poles (-7.1186, 0.6407) (-7.241, 0.8373) (-7.4707, 1.1897) (-7.5978, 1.362) knots 0 0 0 1 2 2 2
  spline S126 degree 2 poles (-7.5978, 1.362) (-7.8538, 1.7092) (-8.1876, 1.9922) (-8.3874, 2.0321) knots 0 0 0 1 2 2 2
  spline S127 degree 2 poles (-8.3874, 2.0321) (-8.4924, 2.0531) (-8.6627, 2.02) (-8.7249, 1.9716) knots 0 0 0 1 2 2 2
  spline S128 degree 2 poles (-8.7249, 1.9716) (-8.7871, 1.9231) (-8.8682, 1.7798) (-8.8868, 1.687) knots 0 0 0 1 2 2 2
  spline S129 degree 2 poles (-8.8868, 1.687) (-8.9045, 1.5982) (-8.8964, 1.4076) (-8.8787, 1.318) knots 0 0 0 1 2 2 2
  spline S130 degree 2 poles (-8.8787, 1.318) (-8.8646, 1.2417) (-8.8101, 1.0944) (-8.7899, 1.0484) knots 0 0 0 1 2 2 2
  line L78 (-8.7899, 1.0484) -> (-8.7935, 1.0302)
  line L79 (-8.7935, 1.0302) -> (-9.1487, 1.1013)
  spline S131 degree 2 poles (-9.1487, 1.1013) (-9.1786, 1.2143) (-9.2036, 1.6034) (-9.1705, 1.7689) knots 0 0 0 1 2 2 2
  spline S132 degree 2 poles (-9.1705, 1.7689) (-9.1007, 2.1181) (-8.6526, 2.4378) (-8.3378, 2.3749) knots 0 0 0 1 2 2 2
  spline S133 degree 2 poles (-8.3378, 2.3749) (-8.1904, 2.3454) (-7.9579, 2.2275) (-7.8651, 2.146) knots 0 0 0 1 2 2 2
  spline S134 degree 2 poles (-7.8651, 2.146) (-7.7682, 2.0636) (-7.5893, 1.8452) (-7.5058, 1.7278) knots 0 0 0 1 2 2 2
  spline S135 degree 2 poles (-7.5058, 1.7278) (-7.3657, 1.536) (-7.0755, 1.0771) (-6.9915, 0.9406) knots 0 0 0 1 2 2 2
  line L80 (-6.9915, 0.9406) -> (-6.7469, 2.1638)
  line L81 (-6.7469, 2.1638) -> (-6.4583, 2.106)
  spline S136 degree 2 poles (-6.7431, 4.4098) (-6.1363, 4.0954) (-5.7507, 3.4481) (-5.9411, 3.0808) knots 0 0 0 1 2 2 2
  spline S137 degree 2 poles (-5.9411, 3.0808) (-6.1342, 2.708) (-6.8945, 2.6591) (-7.4884, 2.9669) knots 0 0 0 1 2 2 2
  spline S138 degree 2 poles (-7.4884, 2.9669) (-8.0988, 3.2831) (-8.4808, 3.9285) (-8.2895, 4.2977) knots 0 0 0 1 2 2 2
  spline S139 degree 2 poles (-8.2895, 4.2977) (-8.0972, 4.6687) (-7.3316, 4.7147) (-6.7431, 4.4098) knots 0 0 0 1 2 2 2
  spline S140 degree 2 poles (-6.2567, 3.6662) (-6.3454, 3.7679) (-6.6701, 3.9825) (-6.9022, 4.1027) knots 0 0 0 1 2 2 2
  spline S141 degree 2 poles (-6.9022, 4.1027) (-7.1343, 4.223) (-7.495, 4.3635) (-7.6338, 4.3775) knots 0 0 0 1 2 2 2
  spline S142 degree 2 poles (-7.6338, 4.3775) (-7.7726, 4.3915) (-7.9738, 4.294) (-8.0391, 4.1679) knots 0 0 0 1 2 2 2
  spline S143 degree 2 poles (-8.0391, 4.1679) (-8.1045, 4.0418) (-8.0699, 3.8176) (-7.9758, 3.7085) knots 0 0 0 1 2 2 2
  spline S144 degree 2 poles (-7.9758, 3.7085) (-7.8843, 3.6032) (-7.5505, 3.3885) (-7.3293, 3.2739) knots 0 0 0 1 2 2 2
  spline S145 degree 2 poles (-7.3293, 3.2739) (-7.0917, 3.1508) (-6.7586, 3.0152) (-6.6097, 2.9984) knots 0 0 0 1 2 2 2
  spline S146 degree 2 poles (-6.6097, 2.9984) (-6.47, 2.9816) (-6.2596, 3.0789) (-6.1914, 3.2105) knots 0 0 0 1 2 2 2
  spline S147 degree 2 poles (-6.1914, 3.2105) (-6.127, 3.3348) (-6.1616, 3.559) (-6.2567, 3.6662) knots 0 0 0 1 2 2 2
  line L82 (-4.3459, 5.2209) -> (-5.4236, 4.0842)
  line L83 (-5.4236, 4.0842) -> (-5.685, 4.332)
  spline S148 degree 2 poles (-5.685, 4.332) (-5.6839, 4.5635) (-5.6907, 4.9841) (-5.7066, 5.1977) knots 0 0 0 1 2 2 2
  spline S149 degree 2 poles (-5.7066, 5.1977) (-5.7385, 5.6279) (-5.8704, 6.0451) (-6.0183, 6.1853) knots 0 0 0 1 2 2 2
  spline S150 degree 2 poles (-6.0183, 6.1853) (-6.096, 6.259) (-6.2578, 6.3216) (-6.3362, 6.3137) knots 0 0 0 1 2 2 2
  spline S151 degree 2 poles (-6.3362, 6.3137) (-6.4146, 6.3058) (-6.5596, 6.2277) (-6.6247, 6.159) knots 0 0 0 1 2 2 2
  spline S152 degree 2 poles (-6.6247, 6.159) (-6.6871, 6.0933) (-6.7817, 5.9277) (-6.8143, 5.8424) knots 0 0 0 1 2 2 2
  spline S153 degree 2 poles (-6.8143, 5.8424) (-6.843, 5.7702) (-6.8753, 5.6165) (-6.8827, 5.5668) knots 0 0 0 1 2 2 2
  line L84 (-6.8827, 5.5668) -> (-6.8954, 5.5534)
  line L85 (-6.8954, 5.5534) -> (-7.1583, 5.8026)
  spline S154 degree 2 poles (-7.1583, 5.8026) (-7.1235, 5.9142) (-6.9375, 6.2569) (-6.8214, 6.3794) knots 0 0 0 1 2 2 2
  spline S155 degree 2 poles (-6.8214, 6.3794) (-6.5764, 6.6378) (-6.0268, 6.67) (-5.7938, 6.449) knots 0 0 0 1 2 2 2
  spline S156 degree 2 poles (-5.7938, 6.449) (-5.6848, 6.3456) (-5.5507, 6.1221) (-5.5155, 6.0036) knots 0 0 0 1 2 2 2
  spline S157 degree 2 poles (-5.5155, 6.0036) (-5.4773, 5.8823) (-5.4422, 5.6023) (-5.434, 5.4583) knots 0 0 0 1 2 2 2
  spline S158 degree 2 poles (-5.434, 5.4583) (-5.4175, 5.2215) (-5.4161, 4.6784) (-5.4177, 4.5182) knots 0 0 0 1 2 2 2
  line L86 (-5.4177, 4.5182) -> (-4.5595, 5.4234)
  line L87 (-4.5595, 5.4234) -> (-4.3459, 5.2209)
  spline S159 degree 2 poles (-3.113, 6.9501) (-3.0139, 6.7815) (-2.9578, 6.4301) (-2.9955, 6.279) knots 0 0 0 1 2 2 2
  spline S160 degree 2 poles (-2.9955, 6.279) (-3.0337, 6.1205) (-3.217, 5.8719) (-3.3643, 5.7853) knots 0 0 0 1 2 2 2
  spline S161 degree 2 poles (-3.3643, 5.7853) (-3.5116, 5.6987) (-3.8131, 5.6552) (-3.9638, 5.7004) knots 0 0 0 1 2 2 2
  spline S162 degree 2 poles (-3.9638, 5.7004) (-4.1473, 5.7525) (-4.5097, 6.0767) (-4.6807, 6.3677) knots 0 0 0 1 2 2 2
  spline S163 degree 2 poles (-4.6807, 6.3677) (-4.8486, 6.6534) (-5.0016, 7.1819) (-4.9793, 7.4242) knots 0 0 0 1 2 2 2
  spline S164 degree 2 poles (-4.9793, 7.4242) (-4.9585, 7.6609) (-4.6918, 8.0683) (-4.4451, 8.2133) knots 0 0 0 1 2 2 2
  spline S165 degree 2 poles (-4.4451, 8.2133) (-4.3723, 8.2561) (-4.2362, 8.3169) (-4.1789, 8.3291) knots 0 0 0 1 2 2 2
  line L88 (-4.1789, 8.3291) -> (-4.0131, 8.047)
  line L89 (-4.0131, 8.047) -> (-4.0255, 8.0397)
  spline S166 degree 2 poles (-4.0255, 8.0397) (-4.0789, 8.037) (-4.2498, 7.9866) (-4.335, 7.9366) knots 0 0 0 1 2 2 2
  spline S167 degree 2 poles (-4.335, 7.9366) (-4.6083, 7.776) (-4.7267, 7.2097) (-4.5459, 6.829) knots 0 0 0 1 2 2 2
  spline S168 degree 2 poles (-4.5459, 6.829) (-4.484, 6.9633) (-4.3109, 7.1724) (-4.1796, 7.2496) knots 0 0 0 1 2 2 2
  spline S169 degree 2 poles (-4.1796, 7.2496) (-4.0518, 7.3247) (-3.8299, 7.3859) (-3.6793, 7.3693) knots 0 0 0 1 2 2 2
  spline S170 degree 2 poles (-3.6793, 7.3693) (-3.5054, 7.3497) (-3.2235, 7.1382) (-3.113, 6.9501) knots 0 0 0 1 2 2 2
  spline S171 degree 2 poles (-3.4038, 6.7625) (-3.4831, 6.8973) (-3.6615, 7.0384) (-3.7771, 7.0564) knots 0 0 0 1 2 2 2
  spline S172 degree 2 poles (-3.7771, 7.0564) (-3.8628, 7.0681) (-4.026, 7.0128) (-4.1023, 6.9679) knots 0 0 0 1 2 2 2
  spline S173 degree 2 poles (-4.1023, 6.9679) (-4.2053, 6.9074) (-4.3622, 6.7316) (-4.4218, 6.6178) knots 0 0 0 1 2 2 2
  spline S174 degree 2 poles (-4.4218, 6.6178) (-4.4048, 6.5848) (-4.3729, 6.5224) (-4.3458, 6.4762) knots 0 0 0 1 2 2 2
  spline S175 degree 2 poles (-4.3458, 6.4762) (-4.2123, 6.2491) (-3.9598, 6.0226) (-3.8496, 5.9895) knots 0 0 0 1 2 2 2
  spline S176 degree 2 poles (-3.8496, 5.9895) (-3.7468, 5.9568) (-3.5796, 5.9811) (-3.5033, 6.0259) knots 0 0 0 1 2 2 2
  spline S177 degree 2 poles (-3.5033, 6.0259) (-3.3259, 6.1302) (-3.2557, 6.5105) (-3.4038, 6.7625) knots 0 0 0 1 2 2 2
  dimension "d28" = 22
  constraints: 1 centre point, 1 coincident, 1 other
  measures "d28" diameter of A0
extrude "Extrusion4" cut sketch "Sketch6" against normal blind 1 contours A0 L35 L36 L37 | S62 S63 L40 L41 L42 S64 S65 S66 L43 L44 L45 L38 L39 S61 A0 | A0 S61 S62 | S48 S40 A0 | A0 S40 S41 S42 S43 L21 L22 S44 S45 S46 L23 L24 S47 S48 | S70 L46 S71 S72 S73 S74 S75 L47 L48 L49 S76 A0 | A0 S76 S77 L50 L51 S67 S68 S69 S70 | A0 L18 L19 L20 | S32 S33 A0 | A0 S33 L11 L12 L13 L14 L15 S34 S35 S32 | S0 S1 S2 S3 S4 S5 L0 L1 S6 S7 S8 S9 S10 S11 S12 S13 L2 L3 S14 S15 A0 | A0 S15 S0 | S17 S18 A0 | A0 S18 S19 S20 S21 L4 S22 S23 S24 L5 L6 S25 S26 S27 L7 L8 L9 S16 S17 | S53 S54 L26 L27 L28 L29 L30 S55 S56 | S82 S83 S84 L53 L54 S85 S86 S87 S88 S89 S90 S91 L55 L56 L57 L58 L59 S92 S93 S94 | L60 L61 L62 L63 | L64 L65 S95 S96 S97 S98 S99 S100 L66 L67 S101 S102 S103 S104 S105 L68 L69 | S106 S107 S108 L70 S109 S110 S111 S112 L71 S113 S114 | L72 L73 L74 L75 | L76 L77 S125 S126 S127 S128 S129 S130 L78 L79 S131 S132 S133 S134 S135 L80 L81 | S136 S137 S138 S139 | L82 L83 S148 S149 S150 S151 S152 S153 L84 L85 S154 S155 S156 S157 S158 L86 L87 | S159 S160 S161 S162 S163 S164 S165 L88 L89 S166 S167 S168 S169 S170
body "Solid1"
